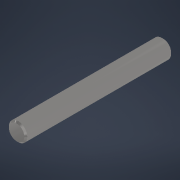
# Autodesk Inventor part: Pin 5x40
Saved by Autodesk Inventor 2022.1 (Build 261234000, 234)
## iProperties
Created: 2021-11-02
Part Number: Pin 5x40
Material: Generisch
Document SubType Name: Modeling
Designer: Rama
Density: 1 g/cm^3
Appearance: Stahl - poliert
Author: Rama
Autodesk Inventor part; units mm, degrees
ref_plane "YZ Plane" through (0, 0, 0) normal (1, 0, 0) x (0, 1, 0)
ref_plane "XZ Plane" through (0, 0, 0) normal (0, 1, 0) x (-1, 0, 0)
ref_plane "XY Plane" through (0, 0, 0) normal (0, 0, 1) x (1, 0, 0)
sketch "Skizze1" plane through (0, 0, 0) normal (0, 0, 1) x (1, 0, 0)
  circle A0 centre (0, 0) radius 2.5
  dimension "d0" = 5
  constraints: 1 centre point, 1 coincident
  measures "d0" diameter of A0
extrude "Extrusion1" add sketch "Skizze1" along normal blind 40
chamfer "Fase1" distance 0.4 angle 45 2 edges at (-2.5, 0, 40) (-2.5, 0, 0)
